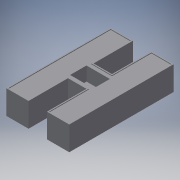
# Autodesk Inventor part: Gebouw Helix V1 Volledig
Saved by Autodesk Inventor 2018.3 (Build 223284000, 284)
## iProperties
Created: 2020-11-24
Part Number: Gebouw Helix V1 Volledig
Material: Generic
Document SubType Name: Modeling
Designer: daanv
Density: 1 g/cm^3
Appearance: Default
Author: daanv
Autodesk Inventor part; units mm, degrees
ref_plane "YZ Plane" through (0, 0, 0) normal (1, 0, 0) x (0, 1, 0)
ref_plane "XZ Plane" through (0, 0, 0) normal (0, 1, 0) x (-1, 0, 0)
ref_plane "XY Plane" through (0, 0, 0) normal (0, 0, 1) x (1, 0, 0)
sketch "Sketch1" plane through (0, 0, 0) normal (0, 0, 1) x (1, 0, 0)
  line L0 (0, 0) -> (0, 90)
  line L1 (0, 90) -> (19.2, 90)
  line L2 (19.2, 90) -> (19.2, 56)
  line L3 (19.2, 56) -> (35.07, 56)
  line L4 (35.07, 56) -> (35.07, 90)
  line L5 (35.07, 90) -> (54.27, 90)
  line L6 (54.27, 90) -> (54.27, 0)
  line L7 (54.27, 0) -> (35.07, 0)
  line L8 (35.07, 0) -> (35.07, 34)
  line L9 (35.07, 34) -> (19.2, 34)
  line L10 (19.2, 34) -> (19.2, 0)
  line L11 (0, 0) -> (19.2, 0)
  dimension "d0" = 90
  dimension "d1" = 19.2
  dimension "d2" = 34
  dimension "d3" = 15.87
  dimension "d4" = 19.2
  dimension "d5" = 34
  dimension "d37" = 22
  constraints: 24 end point, 8 perpendicular, 7 point on line, 1 vertical
  measures "d0" distance of L0.start L0.end
  measures "d1" distance of L0.end L1.end
  measures "d2" distance of L1.end L2.end
  measures "d3" distance of L2.end L3.end
  measures "d4" distance of L4.end L5.end
  measures "d5" distance of L7.end L8.end
  measures "d37" distance between parallel lines of L9 L3
extrude "Extrusion1" add sketch "Sketch1" along normal blind 20.67
sketch "Sketch2" plane through (19.2, 56, 0) normal (0, 1, 0) x (1, 0, 0)
  line L0 (15.87, 0) -> (0, 0) projected
  line L1 (11.39, 0) -> (4.49, 0)
  line L2 (4.49, 0) -> (4.49, -4.29)
  line L3 (4.49, -4.29) -> (11.39, -4.29)
  line L4 (11.39, -4.29) -> (11.39, 0)
  point P0 (-19.2, 0)
  dimension "d8" = 6.9
  dimension "d9" = 4.29
  constraints: 8 end point, 2 parallel, 1 horizontal, 1 perpendicular, 1 point on line
  measures "d8" distance of L3.end L2.end
  measures "d9" distance of L1.end L2.end
extrude "Extrusion2" add sketch "Sketch2" along normal blind 27.15
sketch "Sketch3" plane through (23.69, 56, 4.29) normal (0, 0, 1) x (1, 0, 0)
  line L0 (6.9, 0) -> (0, 0) projected
  line L1 (0, 27.15) -> (6.9, 27.15) projected
  line L2 (0, 0) -> (0, 27.15) projected
  line L3 (6.9, 27.15) -> (9.7769, 2.4369)
  line L4 (6.9, 27.15) -> (31.78, 27.15) construction
  line L5 (9.7769, 2.4369) -> (6.9, 2.4369)
  line L6 (6.9, 0) -> (6.9, 27.15) projected
  line L7 (0, 2.4369) -> (-2.877, 2.4369)
  line L8 (-2.877, 2.4369) -> (0, 27.15)
  point P0 (-23.69, -56)
  dimension "d12" = 24.88
  dimension "d13" = 83.36
  dimension "d14" = 2.877
  constraints: 10 end point, 4 point on line, 2 horizontal, 1 equal length
  measures "d12" distance of L1.end L3.end
  measures "d13" angle of L3 L4
  measures "d14" distance of L7.start L7.end
extrude "Extrusion3" add sketch "Sketch3" against normal blind 4.29
sketch "Sketch4" plane through (19.2, 34, 0) normal (0, -1, 0) x (1, 0, 0)
  line L0 (0, 0) -> (0, 20.67) projected
  line L1 (0, 0) -> (4.49, 0) projected
  line L2 (4.48, 0) -> (11.38, 0)
  line L3 (11.38, 0) -> (11.38, 4.29)
  line L4 (11.38, 4.29) -> (4.48, 4.29)
  line L5 (4.48, 4.29) -> (4.48, 0)
  point P0 (-19.2, 0)
  dimension "d17" = 6.9
  dimension "d18" = 4.29
  dimension "d19" = 4.48
  constraints: 8 end point, 2 parallel, 1 horizontal, 1 perpendicular, 1 point on line
  measures "d17" distance of L4.end L3.end
  measures "d18" distance of L3.end L2.end
  measures "d19" distance between parallel lines of L0 L5
extrude "Extrusion4" add sketch "Sketch4" along normal blind 18.76
sketch "Sketch5" plane through (23.68, 34, 4.29) normal (0, 0, 1) x (1, 0, 0)
  line L0 (0, 0) -> (6.9, 0) projected
  line L1 (0, 0) -> (0, -18.76) projected
  line L2 (6.9, -18.76) -> (0, -18.76) projected
  line L3 (0, -18.76) -> (-2.87, -2.3288)
  line L4 (-4.48, -34) -> (-4.48, 0) projected
  line L5 (-2.87, -2.3288) -> (0, -2.3288)
  line L6 (6.9, 0) -> (6.9, -18.76) projected
  line L7 (6.9, -2.3288) -> (9.777, -2.3288)
  line L8 (9.777, -2.3288) -> (6.9, -18.76)
  point P0 (-23.68, -34)
  dimension "d22" = 16.68
  dimension "d23" = 1.61
  dimension "d24" = 2.877
  constraints: 8 end point, 4 point on line, 1 perpendicular
  measures "d22" distance of L1.end L3.end
  measures "d23" distance from line of L4 L3.end
  measures "d24" distance of L7.start L7.end
extrude "Extrusion5" add sketch "Sketch5" against normal blind 4.29
sketch "Sketch6" plane through (0, 0, 20.67) normal (0, 0, 1) x (1, 0, 0)
  line L0 (0.93, 0.93) -> (0.93, 89.07)
  line L1 (0, 90) -> (19.2, 90) projected
  line L2 (0.93, 89.07) -> (18.27, 89.07)
  line L3 (18.27, 89.07) -> (18.27, 55.07)
  line L4 (18.27, 55.07) -> (36, 55.07)
  line L5 (36, 55.07) -> (36, 89.07)
  line L6 (36, 89.07) -> (53.34, 89.07)
  line L7 (53.34, 89.07) -> (53.34, 0.93)
  line L8 (53.34, 0.93) -> (36, 0.93)
  line L9 (36, 0.93) -> (36, 34.93)
  line L10 (36, 34.93) -> (18.27, 34.93)
  line L11 (18.27, 34.93) -> (18.27, 0.93)
  line L12 (18.27, 0.93) -> (0.93, 0.93)
  line L13 (35.07, 56) -> (19.2, 56) projected
  dimension "d27" = 88.14
  dimension "d28" = 17.34
  dimension "d29" = 34
  dimension "d30" = 17.73
  dimension "d31" = 34
  dimension "d32" = 17.34
  dimension "d33" = 88.14
  dimension "d34" = 34
  dimension "d38" = 0.93
  dimension "d39" = 0.93
  constraints: 24 end point, 7 perpendicular, 7 point on line
  measures "d27" distance of L0.start L0.end
  measures "d28" distance of L0.end L2.end
  measures "d29" distance of L2.end L3.end
  measures "d30" distance of L3.end L4.end
  measures "d31" distance of L4.end L5.end
  measures "d32" distance of L5.end L6.end
  measures "d33" distance of L6.end L7.end
  measures "d34" distance of L8.end L9.end
  measures "d38" distance between parallel lines of L2 L1
  measures "d39" distance between parallel lines of L4 L13
extrude "Extrusion6" cut sketch "Sketch6" against normal blind 0.62
sketch "Sketch7" plane through (0, 0, 20.05) normal (0, 0, 1) x (1, 0, 0)
  line L0 (0.93, 0.93) -> (0.93, 89.07) projected
  line L1 (36, 34.93) -> (18.27, 34.93) projected
  line L2 (53.34, 89.07) -> (53.34, 0.93) projected
  line L3 (18.27, 55.07) -> (36, 55.07) projected
  line L4 (17.08, 52.05) -> (37.18, 52.05)
  line L5 (37.18, 52.05) -> (37.18, 37.95)
  line L6 (37.18, 37.95) -> (17.08, 37.95)
  line L7 (17.08, 37.95) -> (17.08, 52.05)
  point P0 (0, 0)
  dimension "d40" = 14.1
  dimension "d41" = 20.1
  dimension "d42" = 3.02
  dimension "d43" = 3.02
  dimension "d44" = 16.15
  dimension "d45" = 16.16
  constraints: 8 end point, 2 parallel, 1 horizontal, 1 perpendicular
  measures "d40" distance of L4.end L5.end
  measures "d41" distance of L5.end L6.end
  measures "d42" distance between parallel lines of L1 L6
  measures "d43" distance between parallel lines of L3 L4
  measures "d44" distance between parallel lines of L0 L7
  measures "d45" distance between parallel lines of L2 L5
extrude "Extrusion7" cut sketch "Sketch7" against normal blind 12
sketch "Sketch8" plane through (0, 0, 8.05) normal (0, 0, 1) x (1, 0, 0)
  line L0 (17.08, 52.05) -> (37.18, 52.05) projected
  line L1 (17.08, 37.95) -> (17.08, 52.05) projected
  line L2 (21.58, 46.35) -> (32.58, 46.35)
  line L3 (32.58, 46.35) -> (32.58, 43.75)
  line L4 (32.58, 43.75) -> (21.58, 43.75)
  line L5 (21.58, 43.75) -> (21.58, 46.35)
  point P0 (0, 0)
  dimension "d48" = 11
  dimension "d49" = 2.6
  dimension "d50" = 5.7
  dimension "d51" = 4.5
  constraints: 8 end point, 2 parallel, 1 horizontal, 1 perpendicular
  measures "d48" distance of L3.end L4.end
  measures "d49" distance of L2.end L3.end
  measures "d50" distance between parallel lines of L0 L2
  measures "d51" distance between parallel lines of L1 L5
extrude "Extrusion8" cut sketch "Sketch8" against normal up to next
body "Solid1"
